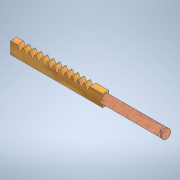
# Autodesk Inventor part: Rack222
Saved by Autodesk Inventor 2022 (Build 260153000, 153)
## iProperties
Created: 2022-06-04
Part Number: Rack222
Material: Generic
Document SubType Name: Modeling
Designer: frede
Density: 1 g/cm^3
Appearance: Default
Author: frede
Autodesk Inventor part; units mm, degrees
ref_plane "YZ Plane" through (0, 0, 0) normal (1, 0, 0) x (0, 1, 0)
ref_plane "XZ Plane" through (0, 0, 0) normal (0, 1, 0) x (-1, 0, 0)
ref_plane "XY Plane" through (0, 0, 0) normal (0, 0, 1) x (1, 0, 0)
sketch "Sketch1" plane through (0, 0, 0) normal (0, 0, 1) x (1, 0, 0)
  spline S0 degree 3 poles (-3.3489, 31.0344) (-3.2669, 30.9208) (-3.1027, 30.6937) (-2.8692, 30.344) (-2.6455, 29.988) (-2.4333, 29.625) (-2.2335, 29.255) (-2.0474, 28.8779) (-1.8767, 28.4936) (-1.7233, 28.102) (-1.5918, 27.7027) (-1.4824, 27.296) (-1.4363, 26.9482) (-1.3713, 26.6753) (-1.3031, 26.4761) (-1.2148, 26.2851) (-1.1055, 26.1048) (-0.9893, 25.973) (-0.8874, 25.8765) (-0.8022, 25.8147) (-0.714, 25.7572) (-0.6186, 25.7128) (-0.5212, 25.6728) (-0.4188, 25.6481) (-0.3154, 25.6283) (-0.1751, 25.6229) (0, 25.6264) (0.1751, 25.6229) (0.3154, 25.6283) (0.4188, 25.6481) (0.5212, 25.6728) (0.6186, 25.7128) (0.714, 25.7572) (0.8022, 25.8147) (0.8874, 25.8765) (0.9893, 25.973) (1.1055, 26.1048) (1.2148, 26.2851) (1.3031, 26.4761) (1.3713, 26.6753) (1.4363, 26.9482) (1.4824, 27.296) (1.5918, 27.7027) (1.7233, 28.102) (1.8767, 28.4936) (2.0474, 28.8779) (2.2335, 29.255) (2.4333, 29.625) (2.6455, 29.988) (2.8692, 30.344) (3.1027, 30.6937) (3.2669, 30.9208) (3.3489, 31.0344) knots 0 0 0 0 0.042039 0.084079 0.126119 0.168158 0.210197 0.252236 0.294274 0.336311 0.378346 0.420376 0.46241 0.483428 0.504444 0.525453 0.546459 0.567453 0.577965 0.588475 0.598984 0.609494 0.620001 0.63051 0.641019 0.651526 0.672547 0.693567 0.704074 0.714583 0.725092 0.735599 0.746109 0.756618 0.767128 0.77764 0.798635 0.81964 0.840649 0.861665 0.882683 0.924717 0.966747 1.008782 1.050819 1.092857 1.134896 1.176935 1.218975 1.261014 1.303054 1.345093 1.345093 1.345093 1.345093
  circle A0 centre (0, 0) radius 25.625 construction
  circle A1 centre (0, 0) radius 27.0162 construction
  circle A2 centre (0, 0) radius 28.75 construction
  line L0 (-3.3489, 31.0344) -> (3.3489, 31.0344)
  point P0 (-3.1048, 30.6922)
  point P1 (-2.8708, 30.3429)
  point P2 (-2.6474, 29.9868)
  point P3 (-2.4354, 29.6238)
  point P4 (-2.2358, 29.2538)
  point P5 (-2.05, 28.8767)
  point P6 (-1.8796, 28.4924)
  point P7 (-1.7269, 28.1007)
  point P8 (-1.5955, 27.7015)
  point P9 (-1.4914, 27.2943)
  point P10 (-1.4177, 26.8804)
  point P11 (-1.368, 26.6762)
  point P12 (-1.2997, 26.4774)
  point P13 (-1.2113, 26.2869)
  point P14 (-1.1005, 26.1085)
  point P15 (-0.9631, 25.9497)
  point P16 (-0.8859, 25.8783)
  point P17 (-0.8017, 25.8154)
  point P18 (-0.7128, 25.7594)
  point P19 (-0.6182, 25.7135)
  point P20 (-0.5203, 25.6754)
  point P21 (-0.4186, 25.6489)
  point P22 (-0.3151, 25.6309)
  point P23 (-0.2102, 25.6249)
  point P24 (0, 25.625)
  point P25 (0.2102, 25.6249)
  point P26 (0.3151, 25.6309)
  point P27 (0.4186, 25.6489)
  point P28 (0.5203, 25.6754)
  point P29 (0.6182, 25.7135)
  point P30 (0.7128, 25.7594)
  point P31 (0.8017, 25.8154)
  point P32 (0.8859, 25.8783)
  point P33 (0.9631, 25.9497)
  point P34 (1.1005, 26.1085)
  point P35 (1.2113, 26.2869)
  point P36 (1.2997, 26.4774)
  point P37 (1.368, 26.6762)
  point P38 (1.4177, 26.8804)
  point P39 (1.4914, 27.2943)
  point P40 (1.5955, 27.7015)
  point P41 (1.7269, 28.1007)
  point P42 (1.8796, 28.4924)
  point P43 (2.05, 28.8767)
  point P44 (2.2358, 29.2538)
  point P45 (2.4354, 29.6238)
  point P46 (2.6474, 29.9868)
  point P47 (2.8708, 30.3429)
  point P48 (3.1048, 30.6922)
  constraints: 3 centre point, 2 end point, 2 horizontal, 106 other
sketch "Sketch2" plane through (0, 0, 0) normal (0, 0, 1) x (1, 0, 0)
  line L0 (-12.3489, 15.4344) -> (107.6511, 15.4344)
  line L1 (107.6511, 15.4344) -> (107.6511, 31.0344)
  line L2 (107.6511, 31.0344) -> (-12.3489, 31.0344)
  line L3 (-12.3489, 31.0344) -> (-12.3489, 15.4344)
  line L4 (-3.3489, 31.0344) -> (3.3489, 31.0344) projected
  point P0 (0, 0)
  dimension "d7" = 120
  dimension "d8" = 15.6
  dimension "d9" = 9
  constraints: 8 end point, 2 parallel, 1 horizontal, 1 perpendicular, 1 point on line
  measures "d7" distance of L2.end L1.end
  measures "d8" distance of L1.end L0.end
  measures "d9" distance from line of L4.start L3
extrude "Extrusion3" add sketch "Sketch2" against normal blind 8
extrude "Extrusion4" cut sketch "Sketch1" against normal blind 8
pattern_linear "Rectangular Pattern1" count 12 spacing 7.9565 along (1, 0, 0) of "Extrusion4"
sketch "Sketch3" plane through (107.6511, 15.4344, 0) normal (1, 0, 0) x (0, 0, -1)
  line L0 (8, 15.6) -> (0, 15.6) projected
  line L1 (4, 15.6) -> (4, 0)
  line L2 (0.0002, 7.8) -> (7.9998, 7.8)
  line L3 (4, 7.8) -> (-3.8, 7.8)
  line L4 (4, 7.8) -> (11.8, 7.8) construction
  line L5 (0, 0) -> (8, 0) projected
  line L6 (-3.8, 7.8) -> (4, 15.6)
  line L7 (4, 15.6) -> (11.8, 7.8)
  line L8 (11.8, 7.8) -> (4, 0)
  line L9 (4, 0) -> (-3.8, 7.8)
  point P0 (0, -15.4344)
  dimension "d17" = 15.6
  dimension "d18" = 7.8
  dimension "d20" = 7.8
  dimension "d21" = 0
  dimension "d22" = 0
  constraints: 16 end point, 2 collinear, 2 midpoint, 2 parallel, 1 horizontal, 1 perpendicular, 1 vertical
  measures "d17" distance of L1.start L1.end
  measures "d18" distance of L3.start L3.end
  measures "d20" distance from line of L0 L2.start
  measures "d21" angle of L5 L2
  measures "d22" distance from line of L1 L3.start
extrude "Extrusion5" add sketch "Sketch3" along normal blind 75
sketch "Sketch4" plane through (182.6511, 15.4344, 0) normal (1, 0, 0) x (0, 0, -1)
  line L0 (0.3, 11.5) -> (7.7, 11.5)
  line L1 (7.7, 11.5) -> (7.7, 4.1)
  line L2 (7.7, 4.1) -> (0.3, 4.1)
  line L3 (0.3, 4.1) -> (0.3, 11.5)
  point P0 (0, -15.4344)
  point P1 (4, 7.8)
  point P2 (-3.8, 7.8)
  point P3 (4, 15.6)
  point P4 (4, 11.5)
  point P5 (0.3, 7.8)
  dimension "d25" = 7.4
  dimension "d26" = 7.4
  constraints: 8 end point, 2 horizontal alignment, 2 midpoint, 2 parallel, 2 vertical alignment, 1 horizontal, 1 perpendicular
  measures "d25" distance of L1.end L2.end
  measures "d26" distance of L0.end L1.end
extrude "Extrusion6" add sketch "Sketch4" along normal blind 3
sketch "Sketch5" plane through (185.6511, 15.4344, 0) normal (1, 0, 0) x (0, 0, -1)
  circle A0 centre (4, 7.8) radius 5.9
  point P0 (0, -15.4344)
  point P1 (-3.8, 7.8)
  point P2 (4, 15.6)
  dimension "d29" = 11.8
  constraints: 1 centre point, 1 coincident, 1 horizontal alignment, 1 vertical alignment
  measures "d29" diameter of A0
extrude "Extrusion7" add sketch "Sketch5" along normal blind 1
equation "\"Module\" = 2.5"
equation "\"PressureAngle\" = 20deg"
equation "\"UnitProfileClearance\" = 0.25"
equation "\"UnitRoundRadius\" = 0.35"
equation "\"HeadDiameter\" = 62.42917"
equation "\"RootDiameter\" = 51.25"
equation "\"BaseDiameter\" = 54.03233"
equation "\"PitchDiameter\" = 57.5"
equation "\"HelixAngle\" = 0"
equation "\"UnitCorrection\" = 0"
equation "\"UnitAddendumModification\" = 0.014165"
equation "\"CircularPitch\" = 7.853982"
equation "\"UnitBacklashShift\" = 0"
equation "\"TotalToolShift\" = 0"
equation "\"IsInternal\" = 0"
body "Solid2"
